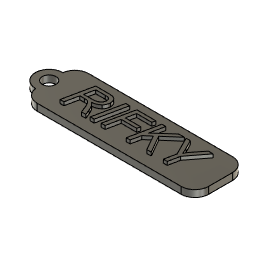
keychain (Autodesk Fusion 360 design; units mm, degrees)
Autodesk Fusion 360 part; units mm, degrees
sketch "Sketch1" plane through (0, 0, 0) normal (0, 0, 1) x (1, 0, 0)
  line L0 (4, 0) -> (46, 0)
  line L1 (50, 4) -> (50, 11)
  line L2 (46, 15) -> (4, 15)
  circle A0 centre (0, 7.5) radius 2
  arc A1 (4, 15) -> (0.0314, 11.4999) centre (4, 11) ccw
  arc A2 (0.0314, 3.5001) -> (4, 0) centre (4, 4) ccw
  arc A3 (50, 11) -> (46, 15) centre (46, 11) ccw
  arc A4 (46, 0) -> (50, 4) centre (46, 4) ccw
  arc A5 (0.0314, 11.4999) -> (0.0314, 3.5001) centre (0, 7.5) ccw
  dimension "d1" = 4
  dimension "d2" = 8
  dimension "d3" = 4
  dimension "d4" = 4
  dimension "d5" = 4
  dimension "d6" = 4
  constraint horizontal L0
  constraint vertical L1
  constraint horizontal L2
  constraint concentric A0 A5
  constraint tangent L2 A1
  constraint tangent L0 A2
  constraint tangent L1 A3
  constraint tangent L2 A3
  constraint tangent L0 A4
  constraint tangent L1 A4
  measures "d1" diameter of A0
  measures "d2" diameter of A5
  measures "d3" radius of A1
  measures "d4" radius of A2
  measures "d5" radius of A3
  measures "d6" radius of A4
extrude "Extrude1" add sketch "Sketch1" along normal blind 2
sketch "Sketch2" plane through (0, 0, 2) normal (0, 0, 1) x (-1, 0, 0)
  circle A0 centre (0, -7.5) radius 2
  arc A1 (-0.0314, -11.4999) -> (-0.0314, -3.5001) centre (0, -7.5) ccw
  arc A2 (-0.0314, -3.5001) -> (-4, 0) centre (-4, -4) ccw
  line L0 (-4, 0) -> (-46, 0)
  arc A3 (-46, 0) -> (-50, -4) centre (-46, -4) ccw
  line L1 (-50, -4) -> (-50, -11)
  arc A4 (-50, -11) -> (-46, -15) centre (-46, -11) ccw
  line L2 (-46, -15) -> (-4, -15)
  arc A5 (-4, -15) -> (-0.0314, -11.4999) centre (-4, -11) ccw
  line L3 (-7.3824, -3.2685) -> (-43.4293, -3.2685) construction
  line L4 (-43.4293, -3.2685) -> (-43.4293, -15.2685) construction
  line L5 (-43.4293, -15.2685) -> (-7.3824, -15.2685) construction
  line L6 (-7.3824, -15.2685) -> (-7.3824, -3.2685) construction
  text T0 "RIFKY" font "Arial" height 12 italic align ink ink in box 0 x 0 at (-7.3824, -3.2685) x (-1, 0) y (0, -1) spacing 1 kerned height is em
  constraint perpendicular L3 L4
  constraint parallel L3 L5
  constraint parallel L4 L6
extrude "Extrude2" add sketch "Sketch2" along normal blind 1 text T0
